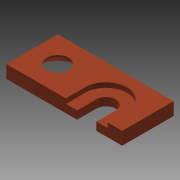
# Autodesk Inventor part: 13_1087_036
Saved by Autodesk Inventor 2014 (Build 180170000, 170)
## iProperties
Created: 2013-09-20
Part Number: 13_1087_036
Material: Allgemein
Document SubType Name: Modeling
Designer: vogel
Density: 1 g/cm^3
Appearance: Kupfer - satiniert
Author: vogel
Autodesk Inventor part; units mm, degrees
ref_plane "YZ Plane" through (0, 0, 0) normal (1, 0, 0) x (0, 1, 0)
ref_plane "XZ Plane" through (0, 0, 0) normal (0, 1, 0) x (-1, 0, 0)
ref_plane "XY Plane" through (0, 0, 0) normal (0, 0, 1) x (1, 0, 0)
sketch "Skizze1" plane through (0, 0, 0) normal (0, 0, 1) x (1, 0, 0)
  line L0 (-21.6, 0) -> (3.6, 0) projected
  line L1 (0, -1.6) -> (0, 9.6) projected
  line L2 (0, 0) -> (-18, 0)
  line L3 (-18, 0) -> (-18, 8)
  line L4 (-18, 8) -> (0, 8)
  line L5 (0, 8) -> (0, 0)
  dimension "d0" = 8
  dimension "d1" = 18
  constraints: 8 end point, 2 parallel, 1 horizontal, 1 perpendicular
  measures "d0" distance of L4.end L2.start
  measures "d1" distance of L2.start L2.end
extrude "Extrusion1" add sketch "Skizze1" along normal blind 2
sketch "Skizze2" plane through (0, 0, 2) normal (0, 0, 1) x (1, 0, 0)
  line L0 (-18, 0) -> (0, 0) projected
  line L1 (0, 0) -> (0, 8) projected
  point P0 (-5.5, 3)
  dimension "d4" = 5.5
  dimension "d5" = 3
  measures "d4" distance from line of point (-5.5, 3) L1
  measures "d5" distance from line of point (-5.5, 3) L0
hole "Bohrung1" at (-5.5, 3, 2) direction (0, 0, -1) diameter 3 depth 8 tip angle 118
sketch "Skizze3" plane through (0, 0, 2) normal (0, 0, 1) x (1, 0, 0)
  circle A0 centre (-5.5, 3) radius 1.5 projected
  line L0 (-18, 0) -> (0, 0) projected
  arc A1 (-2.25, 3) -> (-8.75, 3) centre (-5.5, 3) ccw
  line L1 (-8.75, 3) -> (-8.75, 0)
  line L2 (-2.25, 3) -> (-2.25, 0)
  dimension "d13" = 6.5
  constraints: 4 end point, 2 point on circle, 2 point on line, 2 tangent, 1 centre point, 1 coincident, 1 parallel, 1 perpendicular
  measures "d13" diameter of A1
extrude "Extrusion2" cut sketch "Skizze3" against normal blind 0.75
sketch "Skizze4" plane through (0, 0, 1.25) normal (0, 0, 1) x (1, 0, 0)
  circle A0 centre (-5.5, 3) radius 1.5 projected
  line L0 (-2.25, 0) -> (-8.75, 0) projected
  line L1 (-7, 3) -> (-7, 0)
  line L2 (-4, 3) -> (-4, 0)
  point P0 (0, 0)
  constraints: 4 end point, 2 perpendicular, 2 point on circle, 2 point on line, 2 tangent
extrude "Extrusion3" cut sketch "Skizze4" against normal through all contours L2 L0 L1 A0
sketch "Skizze5" plane through (0, 0, 0) normal (0, 0, -1) x (-1, 0, 0)
  line L0 (7, 0) -> (18, 0) projected
  line L1 (18, 0) -> (18, 8) projected
  arc A0 (8.75, 3) -> (2.25, 3) centre (5.5, 3) ccw projected
  point P0 (14, 4)
  dimension "d18" = 4
  dimension "d19" = 4
  measures "d18" distance from line of point (14, 4) L0
  measures "d19" distance from line of L1 point (14, 4)
hole "Bohrung2" at (-14, 4, 0) direction (0, 0, 1) diameter 3.4 end through all countersink diameter 6.9 countersink angle 90
